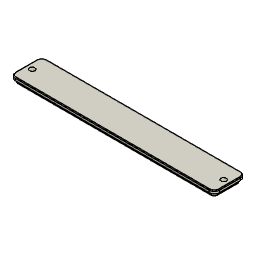
Front Vent -  Blank (Autodesk Fusion 360 design; units mm, degrees)
Autodesk Fusion 360 part; units mm, degrees
sketch "Sketch1" plane through (0, 0, 0) normal (0, 0, 1) x (1, 0, 0)
  line L0 (-84.9, 11.9) -> (84.9, 11.9)
  line L1 (84.9, 11.9) -> (84.9, -11.9)
  line L2 (84.9, -11.9) -> (-84.9, -11.9)
  line L3 (-84.9, -11.9) -> (-84.9, 11.9)
  circle A0 centre (-81.9, 8.9) radius 3
  circle A1 centre (-81.9, -8.9) radius 3
  circle A2 centre (81.9, 8.9) radius 3
  circle A3 centre (81.9, -8.9) radius 3
  line L4 (-107.1873, 0) -> (-105, 0)
  line L5 (-105, 0) -> (105, 0) construction
  circle A4 centre (-81, 0) radius 2.2
  circle A5 centre (81, 0) radius 2.2
  dimension "d21" = 169.8
  dimension "d22" = 84.9
  dimension "d23" = 23.8
  dimension "d24" = 11.9
  dimension "d25" = 6
  dimension "d26" = 6
  dimension "d27" = 6
  dimension "d28" = 6
  dimension "d29" = 210
  dimension "d30" = 4.4
  dimension "d31" = 4.4
  dimension "d32" = 3.9
  dimension "d33" = 3.9
  constraint horizontal L0
  constraint vertical L1
  constraint horizontal L2
  constraint vertical L3
  constraint tangent L0 A0
  constraint tangent L3 A0
  constraint tangent L2 A1
  constraint tangent L3 A1
  constraint tangent L2 A3
  constraint tangent L0 A2
  constraint tangent L1 A2
  constraint tangent L1 A3
  constraint parallel L2 L4
  constraint parallel L2 L5
  constraint midpoint origin L5
  constraint coincident L5 A4.centre
  constraint coincident L5 A5.centre
  measures "d21" distance of L0.start L0.end
  measures "d22" distance of origin L3
  measures "d23" distance of L0.start L2.end
  measures "d24" distance of origin L0
  measures "d25" diameter of A0
  measures "d26" diameter of A1
  measures "d27" diameter of A2
  measures "d28" diameter of A3
  measures "d29" distance of L4.end L5.end
  measures "d30" diameter of A4
  measures "d31" diameter of A5
  measures "d32" distance of L3 A4.centre
  measures "d33" distance of L1 A5.centre
extrude "Extrude1" add sketch "Sketch1" along normal blind 2.8 contours L0 L1 L2 L3 A0 A1 A2 A3 | A0 | A2 | A1 | A3
sketch "Sketch2" plane through (0, 0, 2.8) normal (0, 0, 1) x (-1, 0, 0)
  circle A0 centre (81, 0) radius 2.2
  circle A1 centre (-81, 0) radius 2.2
  arc A2 (81.9, -11.9) -> (84.9, -8.9) centre (81.9, -8.9) ccw
  line L0 (84.9, -8.9) -> (84.9, 8.9)
  arc A3 (84.9, 8.9) -> (81.9, 11.9) centre (81.9, 8.9) ccw
  line L1 (81.9, 11.9) -> (-81.9, 11.9)
  arc A4 (-81.9, 11.9) -> (-84.9, 8.9) centre (-81.9, 8.9) ccw
  line L2 (-84.9, 8.9) -> (-84.9, -8.9)
  arc A5 (-84.9, -8.9) -> (-81.9, -11.9) centre (-81.9, -8.9) ccw
  line L3 (-81.9, -11.9) -> (81.9, -11.9)
  line L4 (-81.9, -13.3) -> (81.9, -13.3)
  arc A6 (81.9, -13.3) -> (86.3, -8.9) centre (81.9, -8.9) ccw
  line L5 (86.3, -8.9) -> (86.3, 8.9)
  arc A7 (86.3, 8.9) -> (81.9, 13.3) centre (81.9, 8.9) ccw
  line L6 (81.9, 13.3) -> (-81.9, 13.3)
  arc A8 (-81.9, 13.3) -> (-86.3, 8.9) centre (-81.9, 8.9) ccw
  line L7 (-86.3, 8.9) -> (-86.3, -8.9)
  arc A9 (-86.3, -8.9) -> (-81.9, -13.3) centre (-81.9, -8.9) ccw
  dimension "d36" = 1.4
extrude "Extrude2" add sketch "Sketch2" along normal blind 2.4 contours A2 L0 A3 L1 A4 L2 A5 L3 | L4 A6 L5 A7 L6 A8 L7 A9
chamfer "Chamfer1" distance 0.6 angle 45 8 edges at (86.3, 0, 5.2) (85.0113, 12.0113, 5.2) (0, 13.3, 5.2) (-85.0113, 12.0113, 5.2) (-86.3, 0, 5.2) (-85.0113, -12.0113, 5.2) (0, -13.3, 5.2) (85.0113, -12.0113, 5.2)
sketch "Sketch4" plane through (-1.7827, -2.3697, 0) normal (0, 0, -1) x (1, 0, 0)
  circle A0 centre (-79.2173, -2.3697) radius 2.2
  circle A1 centre (82.7827, -2.3697) radius 2.2
  arc A2 (-83.1173, -11.2697) -> (-80.1173, -14.2697) centre (-80.1173, -11.2697) ccw
  line L0 (-80.1173, -14.2697) -> (83.6827, -14.2697)
  arc A3 (83.6827, -14.2697) -> (86.6827, -11.2697) centre (83.6827, -11.2697) ccw
  line L1 (86.6827, -11.2697) -> (86.6827, 6.5303)
  arc A4 (86.6827, 6.5303) -> (83.6827, 9.5303) centre (83.6827, 6.5303) ccw
  line L2 (83.6827, 9.5303) -> (-80.1173, 9.5303)
  arc A5 (-80.1173, 9.5303) -> (-83.1173, 6.5303) centre (-80.1173, 6.5303) ccw
  line L3 (-83.1173, 6.5303) -> (-83.1173, -11.2697)
  line L4 (-82.6173, 6.5303) -> (-82.6173, -11.2697)
  arc A6 (-82.6173, -11.2697) -> (-80.1173, -13.7697) centre (-80.1173, -11.2697) ccw
  line L5 (-80.1173, -13.7697) -> (83.6827, -13.7697)
  arc A7 (83.6827, -13.7697) -> (86.1827, -11.2697) centre (83.6827, -11.2697) ccw
  line L6 (86.1827, -11.2697) -> (86.1827, 6.5303)
  arc A8 (86.1827, 6.5303) -> (83.6827, 9.0303) centre (83.6827, 6.5303) ccw
  line L7 (83.6827, 9.0303) -> (-80.1173, 9.0303)
  arc A9 (-80.1173, 9.0303) -> (-82.6173, 6.5303) centre (-80.1173, 6.5303) ccw
  dimension "d44" = -0.5
extrude "Extrude4" cut sketch "Sketch4" against normal up to surface (2.8 mm away) contours A2 L0 A3 L1 A4 L2 A5 L3
equation "d22 = d21 / 2"
equation "d24 = d23 / 2"
equation "d26 = d25"
equation "d27 = d25"
equation "d28 = d25"
equation "d33 = d32"
